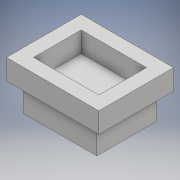
# Autodesk Inventor part: button
Saved by Autodesk Inventor 2017 (Build 210142000, 142)
## iProperties
Part Number: button
Material: Типовые
Document SubType Name: Modeling
Designer: roman
Density: 1 g/cm^3
Appearance: По умолчанию
Author: roman
Autodesk Inventor part; units mm, degrees
ref_plane "YZ Plane" through (0, 0, 0) normal (1, 0, 0) x (0, 1, 0)
ref_plane "XZ Plane" through (0, 0, 0) normal (0, 1, 0) x (-1, 0, 0)
ref_plane "XY Plane" through (0, 0, 0) normal (0, 0, 1) x (1, 0, 0)
sketch "Эскиз1" plane through (0, 0, 0) normal (0, 0, 1) x (1, 0, 0)
  line L0 (0, 0) -> (5.4, 0)
  line L1 (5.4, 0) -> (5.4, 4.4)
  line L2 (5.4, 4.4) -> (0, 4.4)
  line L3 (0, 4.4) -> (0, 0)
  dimension "d0" = 5.4
  dimension "d1" = 4.4
  constraints: 8 end point, 2 parallel, 1 horizontal, 1 perpendicular
  measures "d0" distance of L2.end L1.end
  measures "d1" distance of L1.end L0.end
extrude "Выдавливание1" add sketch "Эскиз1" along normal blind 2
sketch "Эскиз2" plane through (0, 0, 2) normal (0, 0, 1) x (1, 0, 0)
  line L0 (0, 0) -> (5.4, 0) projected
  line L1 (5.4, 0) -> (5.4, 4.4) projected
  line L2 (5.4, 4.4) -> (0, 4.4) projected
  line L3 (0, 4.4) -> (0, 0) projected
  line L4 (0.3, 3.95) -> (5.1, 3.95)
  line L5 (5.1, 3.95) -> (5.1, 0.45)
  line L6 (5.1, 0.45) -> (0.3, 0.45)
  line L7 (0.3, 0.45) -> (0.3, 3.95)
  line L8 (-0.7, 4.95) -> (6.1, 4.95)
  line L9 (6.1, 4.95) -> (6.1, -0.55)
  line L10 (6.1, -0.55) -> (-0.7, -0.55)
  line L11 (-0.7, -0.55) -> (-0.7, 4.95)
  dimension "d4" = 4.8
  dimension "d5" = 3.5
  dimension "d6" = 5.4
  dimension "d7" = 4.4
  dimension "d8" = 0.3
  dimension "d9" = 0.45
  dimension "d12" = 1
  dimension "d13" = 1
  dimension "d14" = 1
  dimension "d15" = 1
  constraints: 16 end point, 4 parallel, 2 horizontal, 2 perpendicular
  measures "d4" distance of L5.end L6.end
  measures "d5" distance of L4.end L5.end
  measures "d6" distance of L0.start L0.end
  measures "d7" distance of L2.end L0.start
  measures "d8" distance between parallel lines of L3 L7
  measures "d9" distance between parallel lines of L4 L2
  measures "d12" distance between parallel lines of L9 L5
  measures "d13" distance between parallel lines of L4 L8
  measures "d14" distance between parallel lines of L11 L7
  measures "d15" distance between parallel lines of L10 L6
extrude "Выдавливание3" add sketch "Эскиз2" along normal blind 1.5 contours L3 L2 L1 L0 | L8 L9 L10 L11
equation "\"d8\" = -0.5 * d4 + 0.5 * d6"
equation "\"d9\" = -0.5 * d5 + 0.5 * d7"
equation "\"d13\" = d12"
equation "\"d14\" = d12"
equation "\"d15\" = d12"
